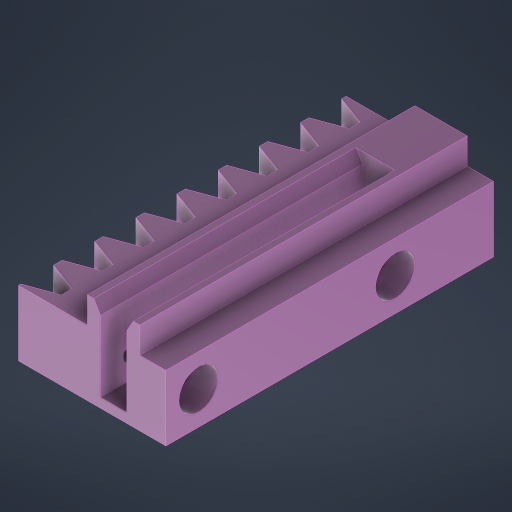
# Autodesk Inventor part: Shaft_V3
Saved by Autodesk Inventor 2024.1 (Build 281209000, 209)
## iProperties
Created: 2023-05-18
Part Number: Shaft_V3
Material: ABS Plastic
Document SubType Name: Modeling
Designer: jaege
Density: 1.06 g/cm^3
Appearance: Smooth - Purple
Mass: 10.7829 g
Surface Area: 60.4361 cm^2
Volume: 10.1725 cm^3
Author: jaege
## iProperties of the stored document Shaft_V3_3DPrint.ipt
Created: 2023-05-19
Part Number: Shaft_V3_3DPrint
Material: Generic
Document SubType Name: Modeling
Designer: jaege
Density: 1 g/cm^3
Appearance: Default
Author: jaege
Autodesk Inventor part; units mm, degrees
ref_plane "YZ Plane" through (0, 0, 0) normal (1, 0, 0) x (0, 1, 0)
ref_plane "XZ Plane" through (0, 0, 0) normal (0, 1, 0) x (-1, 0, 0)
ref_plane "XY Plane" through (0, 0, 0) normal (0, 0, 1) x (1, 0, 0)
sketch "Front" plane through (0, 0, 0) normal (0, 0, 1) x (1, 0, 0)
  line L0 (-9, -5) -> (-3, -5)
  line L1 (9, -5) -> (9, 5)
  line L2 (9, 5) -> (-9, 5)
  line L3 (-9, 5) -> (-9, -5) construction
  line L4 (-9, -5) -> (9, 5) construction
  line L5 (9, -5) -> (-9, 5) construction
  line L6 (-9, 5) -> (-13.5, 5)
  line L7 (-13.5, 5) -> (-13.5, -5)
  line L8 (-13.5, -5) -> (-9, -5)
  line L9 (-9, -5) -> (-9, 5) construction
  line L10 (-3, -5) -> (5, -5) construction
  line L11 (5, -5) -> (5, -9)
  line L12 (5, -9) -> (3, -9)
  line L13 (-3, -9) -> (-3, -5)
  line L14 (-3, -5) -> (5, -5) construction
  line L15 (5, -5) -> (9, -5)
  line L16 (-1, -9) -> (3, -9) construction
  line L17 (3, -9) -> (3, 3.55)
  line L18 (3, 3.55) -> (-1, 3.55)
  line L19 (-1, 3.55) -> (-1, -9)
  line L20 (-1, -9) -> (-3, -9)
  line L21 (3, -9) -> (-1, -9) construction
  point P0 (0, 0)
  point P1 (0, 0)
  point P2 (0, 0)
  dimension "d13" = 18
  dimension "d14" = 4.5
  dimension "d15" = 10
  dimension "d16" = 8
  dimension "d17" = 4
  dimension "d18" = 4
  dimension "d19" = 4
  dimension "d20" = 2
  dimension "d21" = 1.45
  constraints: 44 end point, 12 parallel, 6 perpendicular, 3 collinear, 3 midpoint, 1 coincident, 1 horizontal
  measures "d13" distance between parallel lines of L1 L3
  measures "d14" distance of L6.start L6.end
  measures "d15" distance of L15.end L1.end
  measures "d16" distance of L11.end L13.start
  measures "d17" distance of L10.end L11.end
  measures "d18" distance between parallel lines of L1 L11
  measures "d19" distance of L17.end L19.start
  measures "d20" distance between parallel lines of L11 L17
  measures "d21" distance between parallel lines of L2 L18
extrude "Profile" add sketch "Front" along normal mid plane 40
sketch "Sketch3" plane through (0, 0, 20) normal (0, 0, 1) x (1, 0, 0)
  line L0 (-3, -9) -> (-1, -9) projected
  line L1 (-1, -9) -> (3, -9)
  line L2 (-1, 3.55) -> (3, 3.55) projected
  line L3 (-1, -9) -> (-1, 3.55) projected
  line L4 (3, 3.55) -> (3, -9) construction
  line L5 (9, 5) -> (-13.5, 5) projected
  line L6 (-13.5, 5) -> (-13.5, -5) projected
  line L7 (-13.5, -5) -> (-3, -5) projected
  line L8 (-3, -5) -> (-3, -9) projected
  line L9 (-3, -9) -> (-1, -9) projected
  line L10 (-1, -9) -> (-1, 3.55) construction
  line L11 (-1, 3.55) -> (3, 3.55) construction
  line L12 (3, 3.55) -> (3, -9) projected
  line L13 (3, -9) -> (5, -9) projected
  line L14 (5, -9) -> (5, -5) projected
  line L15 (5, -5) -> (9, -5) projected
  line L16 (9, -5) -> (9, 5) projected
  point P0 (0, 0)
  constraints: 2 end point
extrude "Fill slit" add sketch "Sketch3" along normal blind 10
sketch "Sketch6" plane through (-13.5, -5, -20) normal (0, -1, 0) x (1, 0, 0)
  line L0 (0, -5.9213) -> (4.5, -4.2813)
  line L1 (4.5, -4.2813) -> (4.5, -2.5813)
  line L2 (4.5, -2.5813) -> (0, -0.9413)
  line L3 (0, -0.9413) -> (0, 0.3587)
  line L4 (10.5, 0) -> (10.5, 50) projected
  line L5 (0, 0) -> (0, 50) projected
  line L6 (10.5, 0) -> (10.5, 50) projected
  line L7 (0, 50) -> (10.5, 50) projected
  line L8 (0, 0) -> (0, 50) projected
  line L9 (10.5, 0) -> (0, 0) projected
  line L10 (0, 0.3587) -> (4.5, 1.9987)
  line L11 (4.5, 1.9987) -> (4.5, 3.6987)
  line L12 (4.5, 3.6987) -> (0, 5.3387)
  line L13 (0, 5.3387) -> (0, 6.6387)
  line L14 (0, 6.6387) -> (4.5, 8.2787)
  line L15 (4.5, 8.2787) -> (4.5, 9.9787)
  line L16 (4.5, 9.9787) -> (0, 11.6187)
  line L17 (0, 11.6187) -> (0, 12.9187)
  line L18 (0, 12.9187) -> (4.5, 14.5587)
  line L19 (4.5, 14.5587) -> (4.5, 16.2587)
  line L20 (4.5, 16.2587) -> (0, 17.8987)
  line L21 (0, 17.8987) -> (0, 19.1987)
  line L22 (0, 19.1987) -> (4.5, 20.8387)
  line L23 (4.5, 20.8387) -> (4.5, 22.5387)
  line L24 (4.5, 22.5387) -> (0, 24.1787)
  line L25 (0, 24.1787) -> (0, 25.4787)
  line L26 (0, 25.4787) -> (4.5, 27.1187)
  line L27 (4.5, 27.1187) -> (4.5, 28.8187)
  line L28 (4.5, 28.8187) -> (0, 30.4587)
  line L29 (0, 30.4587) -> (0, 31.7587)
  line L30 (0, 31.7587) -> (4.5, 33.3987)
  line L31 (4.5, 33.3987) -> (4.5, 35.0987)
  line L32 (4.5, 35.0987) -> (0, 36.7387)
  line L33 (0, 36.7387) -> (0, 38.0387)
  line L34 (0, 38.0387) -> (4.5, 39.6787)
  line L35 (4.5, 39.6787) -> (4.5, 41.3787)
  line L36 (4.5, 41.3787) -> (0, 43.0187)
  line L37 (0, 43.0187) -> (0, 44.3187)
  line L38 (0, 44.3187) -> (4.5, 45.9587)
  line L39 (4.5, 45.9587) -> (4.5, 47.6587)
  line L40 (4.5, 47.6587) -> (0, 49.2987)
  line L41 (0, 49.2987) -> (0, 50.5987)
  line L42 (0, 50.5987) -> (4.5, 52.2387)
  line L43 (4.5, 52.2387) -> (4.5, 53.9387)
  line L44 (4.5, 53.9387) -> (0, 55.5787)
  line L45 (0, 55.5787) -> (0, 56.8787)
  line L46 (0, 56.8787) -> (4.5, 58.5187)
  line L47 (4.5, 58.5187) -> (4.5, 60.2187)
  line L48 (4.5, 60.2187) -> (0, 61.8587)
  line L49 (0, 61.8587) -> (0, 63.1587)
  line L50 (0, 63.1587) -> (4.5, 64.7987)
  line L51 (4.5, 64.7987) -> (4.5, 66.4987)
  line L52 (4.5, 66.4987) -> (0, 68.1387)
  line L53 (0, 68.1387) -> (0, 69.4387)
  line L54 (0, 69.4387) -> (4.5, 71.0787)
  line L55 (4.5, 71.0787) -> (4.5, 72.7787)
  line L56 (4.5, 72.7787) -> (0, 74.4187)
  line L57 (0, 74.4187) -> (0, 75.7187)
  line L58 (0, 75.7187) -> (4.5, 77.3587)
  line L59 (4.5, 77.3587) -> (4.5, 79.0587)
  line L60 (4.5, 79.0587) -> (0, 80.6987)
  line L61 (0, 80.6987) -> (0, 81.9987)
  line L62 (0, 81.9987) -> (4.5, 83.6387)
  line L63 (4.5, 83.6387) -> (4.5, 85.3387)
  line L64 (4.5, 85.3387) -> (0, 86.9787)
  line L65 (0, 86.9787) -> (0, 88.2787)
  line L66 (0, 88.2787) -> (4.5, 89.9187)
  line L67 (4.5, 89.9187) -> (4.5, 91.6187)
  line L68 (4.5, 91.6187) -> (0, 93.2587)
  line L69 (0, 93.2587) -> (0, 94.5587)
  line L70 (0, 94.5587) -> (4.5, 96.1987)
  line L71 (4.5, 96.1987) -> (4.5, 97.8987)
  line L72 (4.5, 97.8987) -> (0, 99.5387)
  line L73 (0, 99.5387) -> (0, 100.8387)
  line L74 (0, 100.8387) -> (4.5, 102.4787)
  line L75 (4.5, 102.4787) -> (4.5, 104.1787)
  line L76 (4.5, 104.1787) -> (0, 105.8187)
  line L77 (0, 105.8187) -> (0, 107.1187)
  line L78 (0, 107.1187) -> (4.5, 108.7587)
  line L79 (4.5, 108.7587) -> (4.5, 110.4587)
  line L80 (4.5, 110.4587) -> (0, 112.0987)
  line L81 (0, 112.0987) -> (0, 113.3987)
  line L82 (0, 113.3987) -> (4.5, 115.0387)
  line L83 (4.5, 115.0387) -> (4.5, 116.7387)
  line L84 (4.5, 116.7387) -> (0, 118.3787)
  line L85 (0, 118.3787) -> (0, 119.6787)
  line L86 (0, 119.6787) -> (4.5, 121.3187)
  line L87 (4.5, 121.3187) -> (4.5, 123.0187)
  line L88 (4.5, 123.0187) -> (0, 124.6587)
  line L89 (0, 124.6587) -> (0, 125.9587)
  line L90 (0, 125.9587) -> (4.5, 127.5987)
  line L91 (4.5, 127.5987) -> (4.5, 129.2987)
  line L92 (4.5, 129.2987) -> (0, 130.9387)
  line L93 (0, 130.9387) -> (0, 132.2387)
  line L94 (0, 132.2387) -> (4.5, 133.8787)
  line L95 (4.5, 133.8787) -> (4.5, 135.5787)
  line L96 (4.5, 135.5787) -> (0, 137.2187)
  line L97 (0, 137.2187) -> (0, 138.5187)
  line L98 (0, 138.5187) -> (4.5, 140.1587)
  line L99 (4.5, 140.1587) -> (4.5, 141.8587)
  line L100 (4.5, 141.8587) -> (0, 143.4987)
  line L101 (0, 143.4987) -> (0, 144.7987)
  line L102 (0, 144.7987) -> (4.5, 146.4387)
  line L103 (4.5, 146.4387) -> (4.5, 148.1387)
  line L104 (4.5, 148.1387) -> (0, 149.7787)
  line L105 (0, 149.7787) -> (0, 151.0787)
  point P0 (13.5, 20)
  point P1 (0, 30.4587)
  point P2 (0, 25.4787)
  point P3 (0, 17.8987)
  point P4 (0, 6.6387)
  point P5 (0.0109, 0)
  point P6 (0, 49.2987)
  point P7 (0, 54.22)
  point P8 (0, 49.24)
  dimension "d56" = 6
  dimension "d57" = 6.28
  dimension "d59" = 1.3
  dimension "d60" = 1.7
  dimension "d64" = 6.28
  constraints: 200 end point, 121 vertical alignment, 49 parallel, 48 collinear, 2 vertical, 1 equal length, 1 other
  measures "d56" distance between parallel lines of L4 L1
  measures "d57" distance of L3.end L0.start
  measures "d59" distance of L2.end L3.end
  measures "d60" distance of L0.end L1.end
  measures "d64" distance of L0.start L10.start
chamfer "Chamfer1" distance 1 angle 60 2 edges at (3, -9, 0) (-1, -9, 0) measured on face at (-1.5, -9, 0) measured on face at (3.5, -9, 0)
extrude "Extrusion4" cut sketch "Sketch6" against normal blind 10 contours L5 L12 L11 L10 | L5 L16 L15 L14 | L40 L39 L38 L5 | L5 L20 L19 L18 | L36 L35 L34 L5 | L5 L24 L23 L22 | L32 L31 L30 L5 | L5 L28 L27 L26
sketch "Sketch7" plane through (9, -5, -20) normal (1, 0, 0) x (0, 0, -1)
  line L0 (-50, 10) -> (0, 10) projected
  line L1 (-50, 0) -> (-50, 10) projected
  line L2 (0, 0) -> (-50, 0) projected
  line L3 (0, 10) -> (0, 0) projected
  point P0 (-20, 5)
  point P1 (-35, 5)
  point P2 (-5, 5)
  dimension "d72" = 30
  dimension "d73" = 5
  constraints: 2 horizontal alignment
  measures "d72" distance of point (-5, 5) point (-35, 5)
  measures "d73" distance from line of L3 point (-5, 5)
hole "Hole2" at (9, 0, 15) at (9, 0, -15) direction (-1, 0, 0) diameter 3.1 depth 12 counterbore diameter 6 counterbore depth 4
